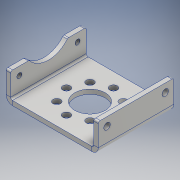
# Autodesk Inventor part: G-ROBOTSアルミブラケットC
Saved by Autodesk Inventor 2017 (Build 210142000, 142)
## iProperties
Created: 2016-11-10
Part Number: G-ROBOTSアルミブラケットC
Material: アルミニウム 6061
Document SubType Name: Sheet Metal
Designer: NN
Density: 2.7 g/cm^3
Flat Pattern Width: 2 cm
Flat Pattern Length: 3.62296 cm
Flat Pattern Area: 7.24591 cm^2
Sheet Metal Rule: Default_mm
Sheet Metal Width: 20.000 mm
Sheet Metal Length: 36.230 mm
Sheet Metal Area: 724.591 mm^2
Appearance: アルミニウム - フラット
Mass: 2.03172 g
Surface Area: 15.0404 cm^2
Volume: 0.752491 cm^3
Author: NN
Autodesk Inventor part; units mm, degrees
ref_plane "YZ Plane" through (0, 0, 0) normal (1, 0, 0) x (0, 1, 0)
ref_plane "XZ Plane" through (0, 0, 0) normal (0, 1, 0) x (-1, 0, 0)
ref_plane "XY Plane" through (0, 0, 0) normal (0, 0, 1) x (1, 0, 0)
sketch "スケッチ1" plane through (0, 0, 0) normal (0, 0, 1) x (1, 0, 0)
  line L0 (11, -10) -> (-11, -10)
  line L1 (-11, -10) -> (-11, 10)
  line L2 (-11, 10) -> (11, 10)
  line L3 (11, 10) -> (11, -10)
  line L4 (11, -10) -> (-11, 10) construction
  line L5 (-11, -10) -> (11, 10) construction
  point P0 (0, 0)
  dimension "d2" = 22
  dimension "d3" = 20
  measures "d2" distance of L0.start L0.end
  measures "d3" distance of L0.end L1.end
extrude "プレート1" add sketch "スケッチ1" along normal blind 1.2
sketch "スケッチ2" plane through (-11, -10, 1.2) normal (-1, 0, 0) x (0, -1, 0)
  line L0 (-20, 0) -> (0, 0)
  line L1 (0, 0) -> (0, 6.5)
  line L2 (0, 6.5) -> (-20, 6.5)
  line L3 (-20, 6.5) -> (-20, 0)
  constraints: 6 end point, 1 horizontal, 1 perpendicular, 1 vertical
edge flange "フランジ1" height 7.7 angle 90 thickness 1.2 bend radius 0.5 thickness toward (-1, 0, 0) relief tear relief width 1.2 relief depth 0.6 corner gap 1.2 corner form 0 edges at (-11, 0, 1.2) (11, 0, 1.2) wall of the first edge with corners at (-11, 10, 1.2) (-11, -10, 1.2) (-11, -10, 7.7) (-11, 10, 7.7)
bend "曲げ1"
corner "コーナー1"
sketch "スケッチ3" plane through (0, 0, 1.2) normal (0, 0, 1) x (1, 0, 0)
  circle A0 centre (0, 0) radius 4.05
  dimension "d15" = 8.1
  constraints: 1 centre point, 1 coincident
  measures "d15" diameter of A0
extrude "押し出し1" cut sketch "スケッチ3" against normal through all
sketch "スケッチ4" plane through (0, 0, 1.2) normal (0, 0, 1) x (1, 0, 0)
  line L0 (0, 0) -> (0, 6.2225)
  circle A0 centre (0, 6.2225) radius 0.9423
  circle A1 centre (-4.4, 4.4) radius 0.9423
  circle A2 centre (-6.2225, 0) radius 0.9423
  circle A3 centre (-4.4, -4.4) radius 0.9423
  circle A4 centre (0, -6.2225) radius 0.9423
  circle A5 centre (4.4, -4.4) radius 0.9423
  circle A6 centre (6.2225, 0) radius 0.9423
  circle A7 centre (4.4, 4.4) radius 0.9423
  dimension "d20" = 360
  dimension "d22" = 8.8
  constraints: 8 centre point, 2 end point, 1 coincident, 1 vertical, 17 other
  measures "d22" distance of A7.centre A1.centre
hole "穴1" at (0, 6.2225, 1.2) at (4.4, 4.4, 1.2) at (6.2225, 0, 1.2) at (4.4, -4.4, 1.2) at (0, -6.2225, 1.2) at (-4.4, -4.4, 1.2) at (-6.2225, 0, 1.2) at (-4.4, 4.4, 1.2) direction (0, 0, -1) diameter 2 end through all
sketch "スケッチ5" plane through (12.2, -10, 7.7) normal (1, 0, 0) x (0, 0, -1)
  line L0 (2.2, 2.3) -> (2.2, 17.7)
  line L1 (6.5, 9) -> (6.5, 11) projected
  line L2 (6.5, 2.7775) -> (6.5, 4.7775) projected
  line L3 (6.5, 9) -> (6.5, 11) projected
  line L4 (6.5, 15.2225) -> (6.5, 17.2225) projected
  line L5 (6.5, 13.4) -> (6.5, 15.4) projected
  line L6 (6.5, 4.6) -> (6.5, 6.6) projected
  line L7 (6.5, 4.6) -> (6.5, 6.6) projected
  line L8 (6.5, 13.4) -> (6.5, 15.4) projected
  line L9 (6.5, 5.95) -> (6.5, 14.05) projected
  line L10 (6.5, 0) -> (6.5, 20) projected
  line L11 (6.5, 20) -> (6.5, 0) projected
  line L12 (7.7, 10) -> (2.2, 10)
  dimension "d30" = 15.4
  dimension "d31" = 4.3
  constraints: 4 end point, 1 midpoint, 1 perpendicular, 1 vertical
  measures "d30" distance of L0.start L0.end
  measures "d31" distance between parallel lines of L0 L11
hole "穴2" at (12.2, 7.7, 5.5) at (12.2, -7.7, 5.5) direction (-1, 0, 0) diameter 1.321 end through all thread size "M1.7x0.35" class "6H" standard "ISO Metric profile"
sketch "スケッチ6" plane through (12.2, -10, 7.7) normal (1, 0, 0) x (0, 0, -1)
  circle A0 centre (2.2, 17.7) radius 0.6605 projected
  circle A1 centre (2.2, 2.3) radius 0.6605 projected
  line L0 (6, 0) -> (6, 20) projected
  line L1 (0, 20) -> (6, 20) projected
  line L2 (0, 0) -> (0, 20) projected
  line L3 (6, 0) -> (0, 0) projected
  point P0 (7.7, 10)
hole "穴3" at (12.2, -7.7, 5.5) at (12.2, 7.7, 5.5) direction (-1, 0, 0) diameter 1.7 depth 10 tip angle 118
sketch "スケッチ7" plane through (-12.2, -10, 7.7) normal (-1, 0, 0) x (0, 0, 1)
  circle A0 centre (-2.2, 17.7) radius 0.6605 projected
  circle A1 centre (-2.2, 2.3) radius 0.6605 projected
  line L0 (-6, 20) -> (-6, 0) projected
  line L1 (0, 0) -> (-6, 0) projected
  line L2 (0, 20) -> (0, 0) projected
  line L3 (-6, 20) -> (0, 20) projected
  line L4 (-6.5, 11) -> (-6.5, 9) projected
  line L5 (-6.5, 4.7775) -> (-6.5, 2.7775) projected
  line L6 (-6.5, 11) -> (-6.5, 9) projected
  line L7 (-6.5, 17.2225) -> (-6.5, 15.2225) projected
  line L8 (-6.5, 15.4) -> (-6.5, 13.4) projected
  line L9 (-6.5, 6.6) -> (-6.5, 4.6) projected
  line L10 (-6.5, 6.6) -> (-6.5, 4.6) projected
  line L11 (-6.5, 15.4) -> (-6.5, 13.4) projected
  line L12 (-6.5, 14.05) -> (-6.5, 5.95) projected
  line L13 (-6.5, 0) -> (-6.5, 20) projected
  line L14 (-6.5, 20) -> (-6.5, 0) projected
  line L15 (-6.5, 10) -> (4, 10)
  circle A2 centre (4, 10) radius 6.5
  point P0 (-7.7, 10)
  dimension "d46" = 10.5
  dimension "d47" = 13
  constraints: 2 end point, 1 centre point, 1 coincident, 1 horizontal, 1 midpoint
  measures "d46" distance of L15.start L15.end
  measures "d47" diameter of A2
extrude "押し出し2" cut sketch "スケッチ7" against normal up to surface (1.2 mm away) contours A2 L2 L15 | L15 L2 A2 | A2 L2
fillet "コーナーR1" radius 0.5 6 edges at (-11.6, -10, 7.7) (11.6, -10, 7.7) (11.6, 10, 7.7) (-11.6, 10, 7.7) (-11.6, -5.1235, 7.7) (-11.6, 5.1235, 7.7)
equation "\"d28\" = Thickness"
equation "\"d5\" = BendReliefWidth"
equation "\"d6\" = BendReliefDepth"
equation "\"d7\" = MinimumRemnant"
equation "\"d8\" = BendRadius"
equation "\"d12\" = CornerReliefSize"
equation "\"d13\" = GapSize"
equation "\"d14\" = JacobiRadiusSize"
equation "\"BendRadius\" = Thickness"
equation "\"BendReliefWidth\" = Thickness"
equation "\"BendReliefDepth\" = 0.5 * Thickness"
equation "\"CornerReliefSize\" = 4 * Thickness"
equation "\"MinimumRemnant\" = 2 * Thickness"
equation "\"TransitionRadius\" = BendRadius"
equation "\"JacobiRadiusSize\" = BendRadius"
equation "\"GapSize\" = Thickness"
equation "\"d4\" = BendRadius"
equation "\"Thickness\" = 1.2"
